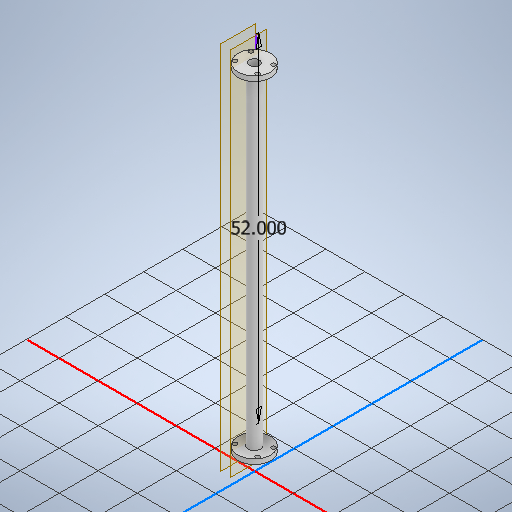
# Autodesk Inventor part: New Metal Pipe
Saved by Autodesk Inventor 2027 (Build 310192000, 192)
## iProperties
Created: 2026-05-22
Part Number: New Metal Pipe
Material: Generic
Document SubType Name: Modeling
Designer: IG2
Density: 1 g/cm^3
Appearance: Default
Author: IG2
Autodesk Inventor part; units mm, degrees
ref_plane "XZ Plane" through (0, 0, 0) normal (0, 1, 0) x (-1, 0, 0)
ref_plane "XY Plane" through (0, 0, 0) normal (0, 0, 1) x (1, 0, 0)
sketch "Sketch1" plane through (0, 0, 0) normal (0, 1, 0) x (-1, 0, 0)
  circle A0 centre (0, 0) radius 23.8125
  circle A1 centre (0, 0) radius 63.5
  dimension "d2" = 127
  dimension "d8" = 47.625
  constraints: 2 centre point, 2 coincident
  measures "d2" diameter of A1
  measures "d8" diameter of A0
extrude "Extrusion1" add sketch "Sketch1" along normal blind 1314.45 contours A0
extrude "Extrusion2" add sketch "Sketch1" along normal blind 19.05
sketch "Sketch3" plane through (0, 1314.45, 0) normal (0, 1, 0) x (1, 0, 0)
  circle A0 centre (0, 0) radius 23.8125 projected
  circle A1 centre (0, 0) radius 63.5
  dimension "d5" = 127
  constraints: 1 centre point, 1 coincident
  measures "d5" diameter of A1
extrude "Extrusion3" add sketch "Sketch3" against normal blind 19.05
sketch "Sketch4" plane through (0, 1314.45, 0) normal (0, 1, 0) x (1, 0, 0)
  circle A0 centre (0, 0) radius 63.5 projected
  line L0 (0, 63.5) -> (0, -63.5)
  line L1 (63.5, 0) -> (-63.5, 0)
  circle A1 centre (44.45, 31.3787) radius 7.9375
  circle A2 centre (0, 0) radius 19.05
  circle A3 centre (44.45, -31.3787) radius 7.9375
  circle A4 centre (-44.45, 31.3787) radius 7.9375
  circle A5 centre (-44.45, -31.3787) radius 7.9375
  dimension "d9" = 38.1
  dimension "d12" = 44.45
  dimension "d13" = 15.875
  constraints: 5 centre point, 4 end point, 4 point on circle, 3 symmetric about line, 1 coincident, 1 midpoint, 1 perpendicular, 1 vertical, 3 other
  measures "d9" diameter of A2
  measures "d12" horizontal distance of A1.centre point (0, 0)
  measures "d13" diameter of A1
extrude "Extrusion4" cut sketch "Sketch4" against normal blind 1314.45 contours A2 L0 L1 | L1 L0 A2 | L0 L1 A2 | A2 L1 L0
extrude "Extrusion5" cut sketch "Sketch4" against normal blind 1314.45 contours A1 | A3 | A4 | A5
ref_plane "Work Plane1" through (-63.5, 0, 0) normal (1, 0, 0) x (0, 1, 0)
sketch "Sketch5" plane through (-63.5, 0, 0) normal (1, 0, 0) x (0, 1, 0)
  line L0 (1314.45, 19.05) -> (0, 19.05) projected
  line L1 (1111.25, 19.05) -> (1111.25, -14.2371)
  line L2 (1314.45, -63.5) -> (1314.45, 63.5) projected
  circle A0 centre (1111.25, 0) radius 6.35
  point P0 (0, 0)
  dimension "d17" = 203.2
  dimension "d18" = 12.7
  constraints: 2 end point, 2 point on line, 1 centre point, 1 vertical
  measures "d17" distance between parallel lines of L2 L1
  measures "d18" diameter of A0
extrude "Extrusion6" cut sketch "Sketch5" along normal blind 44.45
thread "Thread1" size "1/2-13 UNC" class "2B" standard "ANSI Unified Screw Threads" full length
ref_plane "Work Plane2" through (-23.8125, 0, 0) normal (1, 0, 0) x (0, 1, 0)
sketch "Sketch6" plane through (-63.5, 0, 0) normal (1, 0, 0) x (0, 1, 0)
  line L0 (4.6815, -69.7945) -> (23.2887, -69.7945)
  line L1 (23.2887, -69.7945) -> (1344.0887, -69.7945)
  point P0 (0, 0)
  dimension "d23" = 1320.8
  constraints: 4 end point, 1 horizontal, 1 point on line
  measures "d23" distance of L0.end L1.end
body "Solid1"
